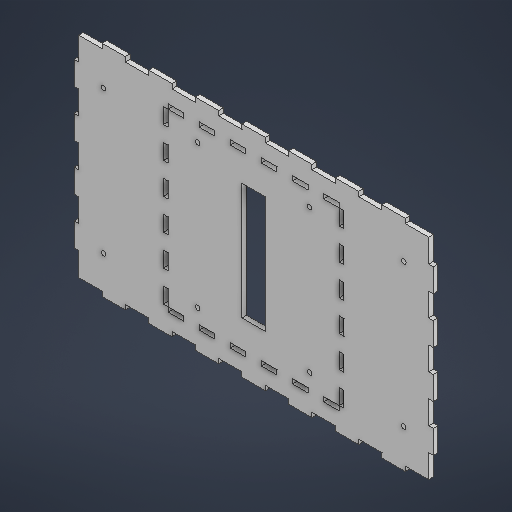
# Autodesk Inventor part: Techo
Saved by Autodesk Inventor 2026 (Build 300175000, 175)
## iProperties
Created: 2026-04-21
Part Number: Techo
Material: Generic
Document SubType Name: Modeling
Designer: juana
Density: 1 g/cm^3
Appearance: Default
Author: juana
Autodesk Inventor part; units mm, degrees
ref_plane "YZ Plane" through (0, 0, 0) normal (1, 0, 0) x (0, 1, 0)
ref_plane "XZ Plane" through (0, 0, 0) normal (0, 1, 0) x (-1, 0, 0)
ref_plane "XY Plane" through (0, 0, 0) normal (0, 0, 1) x (1, 0, 0)
sketch "Sketch1" plane through (0, 0, 0) normal (0, 0, 1) x (1, 0, 0)
  line L0 (0, 135) -> (225, 135)
  line L1 (225, 135) -> (225, 0)
  line L2 (225, 0) -> (0, 0)
  line L3 (0, 0) -> (0, 135)
  dimension "d0" = 135
  dimension "d1" = 225
  constraints: 8 end point, 2 parallel, 1 horizontal, 1 horizontal alignment, 1 perpendicular, 1 vertical alignment
  measures "d0" distance of L0.end L1.end
  measures "d1" distance of L0.start L0.end
extrude "Extrusion1" add sketch "Sketch1" along normal blind 3
sketch "Sketch2" plane through (0, 0, 3) normal (0, 0, 1) x (1, 0, 0)
  line L0 (-3, 120) -> (0, 120)
  line L1 (0, 120) -> (0, 105)
  line L2 (0, 105) -> (-3, 105)
  line L3 (-3, 105) -> (-3, 120)
  line L4 (225, 135) -> (0, 135) projected
  line L5 (-3, 75) -> (-3, 90)
  line L6 (0, 75) -> (-3, 75)
  line L7 (-3, 90) -> (0, 90)
  line L8 (-3, 45) -> (-3, 60)
  line L9 (0, 45) -> (-3, 45)
  line L10 (-3, 60) -> (0, 60)
  line L11 (-3, 15) -> (-3, 30)
  line L12 (0, 15) -> (-3, 15)
  line L13 (-3, 30) -> (0, 30)
  line L14 (225, 105) -> (225, 120)
  line L15 (228, 105) -> (225, 105)
  line L16 (225, 120) -> (228, 120)
  line L17 (225, 75) -> (225, 90)
  line L18 (228, 75) -> (225, 75)
  line L19 (225, 90) -> (228, 90)
  line L20 (225, 45) -> (225, 60)
  line L21 (228, 45) -> (225, 45)
  line L22 (225, 60) -> (228, 60)
  line L23 (225, 15) -> (225, 30)
  line L24 (228, 15) -> (225, 15)
  line L25 (225, 30) -> (228, 30)
  line L26 (228, 120) -> (228, 105)
  line L27 (228, 90) -> (228, 75)
  line L28 (228, 60) -> (228, 45)
  line L29 (228, 30) -> (228, 15)
  line L30 (0, 75) -> (0, 90)
  line L31 (0, 135) -> (0, 0) projected
  line L32 (0, 15) -> (0, 30)
  line L33 (0, 45) -> (0, 60)
  dimension "d4" = 3
  dimension "d5" = 15
  dimension "d6" = 15
  dimension "d9" = 30
  dimension "d12" = 228
  constraints: 64 end point, 5 vertical, 3 collinear, 2 horizontal, 2 parallel, 1 perpendicular, 1 vertical alignment, 50 other
  measures "d4" distance of L0.start L0.end
  measures "d5" distance of L2.end L0.start
  measures "d6" distance from line of L4 L0.end
  measures "d9" distance of L2.end L5.start
  measures "d12" distance of L2.end L14.start
extrude "Extrusion2" add sketch "Sketch2" against normal blind 3
sketch "Sketch3" plane through (0, 0, 3) normal (0, 0, 1) x (1, 0, 0)
  line L0 (225, 135) -> (0, 135) construction
  line L1 (15, 138) -> (30, 138)
  line L2 (30, 138) -> (30, 135)
  line L3 (30, 135) -> (15, 135)
  line L4 (15, 135) -> (15, 138)
  line L5 (60, 135) -> (45, 135)
  line L6 (45, 138) -> (60, 138)
  line L7 (60, 138) -> (60, 135)
  line L8 (45, 135) -> (45, 138)
  line L9 (90, 135) -> (75, 135)
  line L10 (75, 138) -> (90, 138)
  line L11 (90, 138) -> (90, 135)
  line L12 (75, 135) -> (75, 138)
  line L13 (120, 135) -> (105, 135)
  line L14 (105, 138) -> (120, 138)
  line L15 (120, 138) -> (120, 135)
  line L16 (105, 135) -> (105, 138)
  line L17 (150, 135) -> (135, 135)
  line L18 (135, 138) -> (150, 138)
  line L19 (150, 138) -> (150, 135)
  line L20 (135, 135) -> (135, 138)
  line L21 (180, 135) -> (165, 135)
  line L22 (165, 138) -> (180, 138)
  line L23 (180, 138) -> (180, 135)
  line L24 (165, 135) -> (165, 138)
  line L25 (210, 135) -> (195, 135)
  line L26 (195, 138) -> (210, 138)
  line L27 (210, 138) -> (210, 135)
  line L28 (195, 135) -> (195, 138)
  line L29 (0, 135) -> (0, 120) construction
  line L30 (30, -3) -> (15, -3)
  line L31 (15, 0) -> (30, 0)
  line L32 (30, 0) -> (30, -3)
  line L33 (15, -3) -> (15, 0)
  line L34 (60, -3) -> (45, -3)
  line L35 (45, 0) -> (60, 0)
  line L36 (60, 0) -> (60, -3)
  line L37 (45, -3) -> (45, 0)
  line L38 (90, -3) -> (75, -3)
  line L39 (75, 0) -> (90, 0)
  line L40 (90, 0) -> (90, -3)
  line L41 (75, -3) -> (75, 0)
  line L42 (120, -3) -> (105, -3)
  line L43 (105, 0) -> (120, 0)
  line L44 (120, 0) -> (120, -3)
  line L45 (105, -3) -> (105, 0)
  line L46 (150, -3) -> (135, -3)
  line L47 (135, 0) -> (150, 0)
  line L48 (150, 0) -> (150, -3)
  line L49 (135, -3) -> (135, 0)
  line L50 (180, -3) -> (165, -3)
  line L51 (165, 0) -> (180, 0)
  line L52 (180, 0) -> (180, -3)
  line L53 (165, -3) -> (165, 0)
  line L54 (210, -3) -> (195, -3)
  line L55 (195, 0) -> (210, 0)
  line L56 (210, 0) -> (210, -3)
  line L57 (195, -3) -> (195, 0)
  point P0 (0, 0)
  dimension "d17" = 15
  dimension "d18" = 3
  dimension "d19" = 15
  dimension "d22" = 30
  dimension "d25" = 138
  constraints: 112 end point, 2 horizontal, 2 parallel, 1 perpendicular, 1 point on line, 1 vertical, 104 other
  measures "d17" distance of L1.start L1.end
  measures "d18" distance of L1.end L2.end
  measures "d19" distance from line of L0.end L4
  measures "d22" distance of L2.end L5.start
  measures "d25" distance of L2.end L30.start
extrude "Extrusion3" add sketch "Sketch3" against normal blind 3
sketch "Sketch4" plane through (0, 0, 3) normal (0, 0, 1) x (1, 0, 0)
  line L0 (3.5, 120) -> (99, 120) construction
  line L1 (99, 120) -> (99, 15) construction
  line L2 (99, 15) -> (3.5, 15) construction
  line L3 (3.5, 15) -> (3.5, 120) construction
  line L4 (0, 135) -> (0, 120) construction
  line L5 (225, 0) -> (225, 15) construction
  line L6 (0, 135) -> (225, 135) construction
  line L7 (225, 135) -> (225, 0) construction
  line L8 (225, 0) -> (0, 0) construction
  line L9 (0, 0) -> (0, 135) construction
  line L10 (112.5, 0) -> (112.5, 135) construction
  line L11 (45, -3) -> (60, -3) construction
  line L12 (102.5, 120) -> (122.5, 120)
  line L13 (122.5, 120) -> (122.5, 15)
  line L14 (122.5, 15) -> (102.5, 15)
  line L15 (102.5, 15) -> (102.5, 120)
  point P0 (0, 0)
  point P1 (3.5, 67.5)
  point P2 (0, 60)
  point P3 (51.25, 15)
  point P4 (0, 67.5)
  point P5 (16, 113.5)
  point P6 (76.5, 113.5)
  point P7 (16, 21.5)
  point P8 (76.5, 21.5)
  point P9 (112.5, 120)
  point P10 (209, 113.5)
  point P11 (148.5, 113.5)
  point P12 (209, 21.5)
  point P13 (148.5, 21.5)
  dimension "d30" = 95.5
  dimension "d31" = 105
  dimension "d32" = 61.25
  dimension "d33" = 60.5
  dimension "d34" = 12.5
  dimension "d35" = 6.5
  dimension "d36" = 6.5
  dimension "d37" = 20
  constraints: 26 end point, 6 midpoint, 6 parallel, 5 horizontal alignment, 4 symmetric about line, 3 horizontal, 3 perpendicular, 3 vertical alignment
  measures "d30" distance of L0.start L0.end
  measures "d31" distance of L0.end L1.end
  measures "d32" distance from line of L10 point (51.25, 15)
  measures "d33" distance of point (76.5, 113.5) point (16, 113.5)
  measures "d34" distance from line of L3 point (16, 113.5)
  measures "d35" distance from line of L0 point (16, 113.5)
  measures "d36" distance from line of L2 point (16, 21.5)
  measures "d37" distance of L12.start L12.end
hole "Hole1" at (16, 113.5, 3) at (76.5, 113.5, 3) at (16, 21.5, 3) at (76.5, 21.5, 3) at (209, 113.5, 3) at (209, 21.5, 3) at (148.5, 21.5, 3) at (148.5, 113.5, 3) direction (0, 0, -1) diameter 3 end through all
sketch "Sketch5" plane through (0, 0, 3) normal (0, 0, 1) x (1, 0, 0)
  line L0 (0, 135) -> (0, 120) construction
  line L1 (225, 0) -> (225, 15) construction
  line L2 (0, 135) -> (225, 135) construction
  line L3 (225, 135) -> (225, 0) construction
  line L4 (225, 0) -> (0, 0) construction
  line L5 (0, 0) -> (0, 135) construction
  line L6 (105, 105) -> (120, 105)
  line L7 (120, 105) -> (120, 30)
  line L8 (120, 30) -> (105, 30)
  line L9 (105, 30) -> (105, 105)
  point P0 (0, 0)
  point P1 (112.5, 105)
  point P2 (112.5, 135)
  point P3 (105, 67.5)
  point P4 (0, 67.5)
  dimension "d45" = 15
  dimension "d46" = 75
  constraints: 16 end point, 4 midpoint, 4 parallel, 2 horizontal, 2 perpendicular, 1 horizontal alignment, 1 vertical alignment
  measures "d45" distance of L6.start L6.end
  measures "d46" distance of L6.end L7.end
extrude "Extrusion4" cut sketch "Sketch5" against normal blind 3
sketch "Sketch6" plane through (0, 0, 3) normal (0, 0, 1) x (1, 0, 0)
  line L0 (57.5, 122.5) -> (167.5, 122.5) construction
  line L1 (167.5, 122.5) -> (167.5, 12.5) construction
  line L2 (167.5, 12.5) -> (57.5, 12.5) construction
  line L3 (57.5, 12.5) -> (57.5, 122.5) construction
  line L4 (0, 75) -> (0, 60) projected
  line L5 (105, 105) -> (120, 105) construction
  line L6 (57.5, 122.5) -> (54.5, 122.5)
  line L7 (54.5, 122.5) -> (54.5, 112.5)
  line L8 (54.5, 112.5) -> (57.5, 112.5)
  line L9 (57.5, 112.5) -> (57.5, 122.5)
  line L10 (57.5, 102.5) -> (54.5, 102.5)
  line L11 (54.5, 102.5) -> (54.5, 92.5)
  line L12 (54.5, 92.5) -> (57.5, 92.5)
  line L13 (57.5, 92.5) -> (57.5, 102.5)
  line L14 (57.5, 82.5) -> (54.5, 82.5)
  line L15 (54.5, 82.5) -> (54.5, 72.5)
  line L16 (54.5, 72.5) -> (57.5, 72.5)
  line L17 (57.5, 72.5) -> (57.5, 82.5)
  line L18 (57.5, 62.5) -> (54.5, 62.5)
  line L19 (54.5, 62.5) -> (54.5, 52.5)
  line L20 (54.5, 52.5) -> (57.5, 52.5)
  line L21 (57.5, 52.5) -> (57.5, 62.5)
  line L22 (57.5, 42.5) -> (54.5, 42.5)
  line L23 (54.5, 42.5) -> (54.5, 32.5)
  line L24 (54.5, 32.5) -> (57.5, 32.5)
  line L25 (57.5, 32.5) -> (57.5, 42.5)
  line L26 (57.5, 22.5) -> (54.5, 22.5)
  line L27 (54.5, 22.5) -> (54.5, 12.5)
  line L28 (54.5, 12.5) -> (57.5, 12.5)
  line L29 (57.5, 12.5) -> (57.5, 22.5)
  line L30 (170.5, 122.5) -> (167.5, 122.5)
  line L31 (167.5, 122.5) -> (167.5, 112.5)
  line L32 (167.5, 112.5) -> (170.5, 112.5)
  line L33 (170.5, 112.5) -> (170.5, 122.5)
  line L34 (170.5, 102.5) -> (167.5, 102.5)
  line L35 (167.5, 102.5) -> (167.5, 92.5)
  line L36 (167.5, 92.5) -> (170.5, 92.5)
  line L37 (170.5, 92.5) -> (170.5, 102.5)
  line L38 (170.5, 82.5) -> (167.5, 82.5)
  line L39 (167.5, 82.5) -> (167.5, 72.5)
  line L40 (167.5, 72.5) -> (170.5, 72.5)
  line L41 (170.5, 72.5) -> (170.5, 82.5)
  line L42 (170.5, 62.5) -> (167.5, 62.5)
  line L43 (167.5, 62.5) -> (167.5, 52.5)
  line L44 (167.5, 52.5) -> (170.5, 52.5)
  line L45 (170.5, 52.5) -> (170.5, 62.5)
  line L46 (170.5, 42.5) -> (167.5, 42.5)
  line L47 (167.5, 42.5) -> (167.5, 32.5)
  line L48 (167.5, 32.5) -> (170.5, 32.5)
  line L49 (170.5, 32.5) -> (170.5, 42.5)
  line L50 (170.5, 22.5) -> (167.5, 22.5)
  line L51 (167.5, 22.5) -> (167.5, 12.5)
  line L52 (167.5, 12.5) -> (170.5, 12.5)
  line L53 (170.5, 12.5) -> (170.5, 22.5)
  point P0 (0, 0)
  point P1 (57.5, 67.5)
  point P2 (0, 67.5)
  point P3 (112.5, 122.5)
  point P4 (112.5, 105)
  dimension "d49" = 110
  dimension "d50" = 110
  dimension "d51" = 10
  dimension "d52" = 3
  dimension "d55" = 20
  dimension "d58" = 113
  constraints: 104 end point, 4 midpoint, 4 parallel, 3 horizontal, 2 perpendicular, 1 horizontal alignment, 1 vertical, 1 vertical alignment, 88 other
  measures "d49" distance of L1.end L2.end
  measures "d50" distance of L0.end L1.end
  measures "d51" distance of L6.end L7.end
  measures "d52" distance of L0.start L6.end
  measures "d55" distance of L0.start L10.start
  measures "d58" distance of L0.start L30.start
extrude "Extrusion5" cut sketch "Sketch6" against normal blind 3
sketch "Sketch7" plane through (0, 0, 3) normal (0, 0, 1) x (1, 0, 0)
  line L0 (57.5, 112.5) -> (57.5, 122.5) construction
  line L1 (167.5, 12.5) -> (167.5, 22.5) construction
  line L2 (57.5, 122.5) -> (167.5, 122.5) construction
  line L3 (167.5, 122.5) -> (167.5, 12.5) construction
  line L4 (167.5, 12.5) -> (57.5, 12.5) construction
  line L5 (57.5, 12.5) -> (57.5, 122.5) construction
  line L6 (57.5, 122.5) -> (67.5, 122.5)
  line L7 (67.5, 122.5) -> (67.5, 125.5)
  line L8 (67.5, 125.5) -> (57.5, 125.5)
  line L9 (57.5, 125.5) -> (57.5, 122.5)
  line L10 (77.5, 122.5) -> (87.5, 122.5)
  line L11 (87.5, 122.5) -> (87.5, 125.5)
  line L12 (87.5, 125.5) -> (77.5, 125.5)
  line L13 (77.5, 125.5) -> (77.5, 122.5)
  line L14 (97.5, 122.5) -> (107.5, 122.5)
  line L15 (107.5, 122.5) -> (107.5, 125.5)
  line L16 (107.5, 125.5) -> (97.5, 125.5)
  line L17 (97.5, 125.5) -> (97.5, 122.5)
  line L18 (117.5, 122.5) -> (127.5, 122.5)
  line L19 (127.5, 122.5) -> (127.5, 125.5)
  line L20 (127.5, 125.5) -> (117.5, 125.5)
  line L21 (117.5, 125.5) -> (117.5, 122.5)
  line L22 (137.5, 122.5) -> (147.5, 122.5)
  line L23 (147.5, 122.5) -> (147.5, 125.5)
  line L24 (147.5, 125.5) -> (137.5, 125.5)
  line L25 (137.5, 125.5) -> (137.5, 122.5)
  line L26 (157.5, 122.5) -> (167.5, 122.5)
  line L27 (167.5, 122.5) -> (167.5, 125.5)
  line L28 (167.5, 125.5) -> (157.5, 125.5)
  line L29 (157.5, 125.5) -> (157.5, 122.5)
  line L30 (57.5, 9.5) -> (67.5, 9.5)
  line L31 (67.5, 9.5) -> (67.5, 12.5)
  line L32 (67.5, 12.5) -> (57.5, 12.5)
  line L33 (57.5, 12.5) -> (57.5, 9.5)
  line L34 (77.5, 9.5) -> (87.5, 9.5)
  line L35 (87.5, 9.5) -> (87.5, 12.5)
  line L36 (87.5, 12.5) -> (77.5, 12.5)
  line L37 (77.5, 12.5) -> (77.5, 9.5)
  line L38 (97.5, 9.5) -> (107.5, 9.5)
  line L39 (107.5, 9.5) -> (107.5, 12.5)
  line L40 (107.5, 12.5) -> (97.5, 12.5)
  line L41 (97.5, 12.5) -> (97.5, 9.5)
  line L42 (117.5, 9.5) -> (127.5, 9.5)
  line L43 (127.5, 9.5) -> (127.5, 12.5)
  line L44 (127.5, 12.5) -> (117.5, 12.5)
  line L45 (117.5, 12.5) -> (117.5, 9.5)
  line L46 (137.5, 9.5) -> (147.5, 9.5)
  line L47 (147.5, 9.5) -> (147.5, 12.5)
  line L48 (147.5, 12.5) -> (137.5, 12.5)
  line L49 (137.5, 12.5) -> (137.5, 9.5)
  line L50 (157.5, 9.5) -> (167.5, 9.5)
  line L51 (167.5, 9.5) -> (167.5, 12.5)
  line L52 (167.5, 12.5) -> (157.5, 12.5)
  line L53 (157.5, 12.5) -> (157.5, 9.5)
  point P0 (0, 0)
  dimension "d63" = 10
  dimension "d64" = 3
  dimension "d67" = 20
  dimension "d70" = 113
  constraints: 104 end point, 4 parallel, 3 horizontal, 2 perpendicular, 1 vertical, 88 other
  measures "d63" distance of L7.end L8.end
  measures "d64" distance of L8.end L0.end
  measures "d67" distance of L7.end L11.end
  measures "d70" distance of L7.end L31.end
extrude "Extrusion6" cut sketch "Sketch7" against normal blind 3
body "Solid1"
